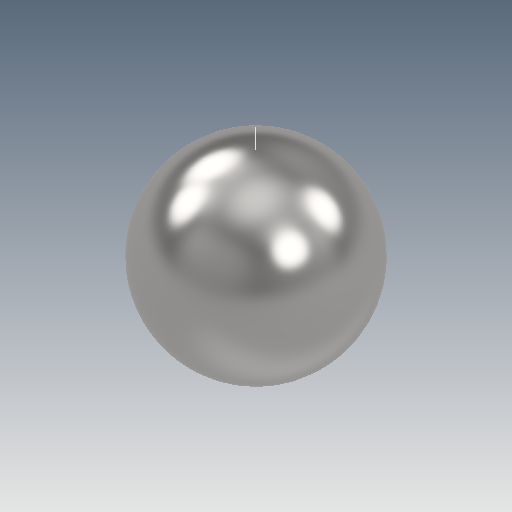
# Autodesk Inventor part: 钢珠
Saved by Autodesk Inventor 2020 (Build 240168000, 168)
## iProperties
Created: 2021-04-21
Part Number: 钢珠
Material: 钢，合金
Document SubType Name: Modeling
Designer: Luorily
Density: 7.73 g/cm^3
Appearance: 半抛光
Author: Luorily
Autodesk Inventor part; units mm, degrees
ref_plane "YZ Plane" through (0, 0, 0) normal (1, 0, 0) x (0, 1, 0)
ref_plane "XZ Plane" through (0, 0, 0) normal (0, 1, 0) x (-1, 0, 0)
ref_plane "XY Plane" through (0, 0, 0) normal (0, 0, 1) x (1, 0, 0)
sketch "草图1" plane through (0, 0, 0) normal (0, 0, 1) x (1, 0, 0)
  arc A0 (6.35, 0) -> (-6.35, 0) centre (0, 0) ccw
  line L0 (6.35, 0) -> (-6.35, 0)
  dimension "d0" = 12.7
  constraints: 2 end point, 2 point on circle, 1 centre point, 1 coincident, 1 horizontal
  measures "d0" diameter of A0
revolve "旋转1" add sketch "草图1" angle 360 about axis through (6.35, 0, 0) along (-1, 0, 0)
